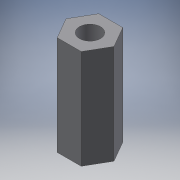
# Autodesk Inventor part: SpacerShiel
Saved by Autodesk Inventor 2017 (Build 210142000, 142)
## iProperties
Created: 2017-12-09
Part Number: SpacerShiel
Material: Generic
Document SubType Name: Modeling
Designer: P. Baesso
Density: 1 g/cm^3
Appearance: Default
Author: P. Baesso
Autodesk Inventor part; units mm, degrees
ref_plane "YZ Plane" through (0, 0, 0) normal (1, 0, 0) x (0, 1, 0)
ref_plane "XZ Plane" through (0, 0, 0) normal (0, 1, 0) x (-1, 0, 0)
ref_plane "XY Plane" through (0, 0, 0) normal (0, 0, 1) x (1, 0, 0)
sketch "Sketch1" plane through (0, 0, 0) normal (0, 0, 1) x (1, 0, 0)
  circle A0 centre (-2.413, 0) radius 2.413 projected
  line L0 (-1.2065, -2.0897) -> (-3.6195, -2.0897)
  line L1 (-3.6195, -2.0897) -> (-4.826, 0)
  line L2 (-4.826, 0) -> (-3.6195, 2.0897)
  line L3 (-3.6195, 2.0897) -> (-1.2065, 2.0897)
  line L4 (-1.2065, 2.0897) -> (0, 0)
  line L5 (0, 0) -> (-1.2065, -2.0897)
  circle A1 centre (-2.413, 0) radius 1.05
  line L6 (-1.913, -3.5) -> (-9.8027, -3.5) projected
  point P0 (0, 0)
  dimension "d0" = 2.1
  constraints: 12 end point, 2 coincident, 1 centre point, 1 parallel, 15 other
  measures "d0" diameter of A1
extrude "Extrusion1" add sketch "Sketch1" against normal blind 10 contours L5 L0 L1 L2 L3 L4
body "Solid1"
